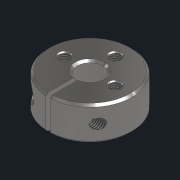
# Autodesk Inventor part: SCSTR6-8b
Saved by Autodesk Inventor 2022 (Build 260153000, 153)
## iProperties
Part Number: SCSTR6-8b
Material: 鋼、炭素鋼
Catalog Web Link: www.cadenas.de
Description: SCST, PSCST, SSCST, SCSTR, PSCSTR, SSCSTR-b-Shaft Collars - 3 Holes/3 Taps
Vendor: MISUMI
Document SubType Name: Modeling
Designer: partserver
Manufacturer: MISUMI
Mass: 15.0833 g
Surface Area: 15.3137 cm^2
Volume: 1.92144 cm^3
Density: 7.85 g/cm^3
Appearance: 半つや出し
Category: PARTsolutions
Company: MISUMI
PSOL_IDENT_0: {$CADENAS_DATA\23d-libs\misumi\metric\03_set_collars\scst\scst_b.prj},209 {VTYP=3D},{NB=SCSTR6-8b},{
PSOL_IDENT_1: LINA=SCSTR6-8},{NN=SCST, PSCST, SSCST, SCSTR, PSCSTR, SSCSTR-b},{DATE=30.06.2021 12:52:04},{GEOMDATE=
PSOL_IDENT_2: 30.10.2015 01:43:51},{VERSION=},{LINEID=220},{WBVAR=TS,MAT,ST,BS},{WBNUMERIC=BS}  {NB=SCSTR6-8b},{LI
PSOL_IDENT_3: NA=SCSTR6-8},{KT=DUMMY},{PN=SCSTR6-8},{TYPE=SCSTR},{TS=3T},{TSALG= '3H' , '3-Hole' , '3T' , '3-Tappe
PSOL_IDENT_4: d' },{TSA= '3H' , '3-Hole', '3T', '3 Tap (Coarse)'},{MAT=S45C},{ST=BO},{STALG= 'BO' , 'Black Oxide'
PSOL_IDENT_5: , 'ENP' , 'Electroless Nickel Plating' },{AC=Hex Socket Head Cap Screw 1 pc.},{ACMAT=4137 Alloy Stee
PSOL_IDENT_6: l},{D=6},{BS=8},{BALG= 8 , 10 },{D1=20},{M=M3},{M3D=3},{DD=3.4},{R=3.00},{W=1.0},{X=6.0},{Y=4},{P=12
PSOL_IDENT_7: },{C=0.5},{S=0.0},{M1=M3},{M13D=3},{L=12}
NB: SCSTR6-8b
NN: SCST, PSCST, SSCST, SCSTR, PSCSTR, SSCSTR-b
NT: Shaft Collars - 3 Holes/3 Taps
NBSYN: $PN.b
LINA: SCSTR6-8
CATALOG: Misumi
PN: SCSTR6-8
TS: 3-Tapped
MAT: 1045 Carbon Steel
ST: Black Oxide
AC: Hex Socket Head Cap Screw 1 pc.
ACMAT: 4137 Alloy Steel
D: 6
BS: 8
D1: 20
M: M3
DD: 3.4
R: 3
W: 1
X: 6
Y: 4
P: 12
C: 0.5
S: 0
M1: M3
SUPPLIER: MISUMI
ARTICLENO: SCSTR6-8b
BOMINFO: SCSTR6-8
CREATOR: CADENAS GmbH
Title: SCSTR6-8
Author: Cadenas PARTsolutions
Comments: Shaft Collars - 3 Holes/3 Taps
Autodesk Inventor part; units mm, degrees
sketch "Sketch_14" plane through (0, 0, 0) normal (1, 0, 0) x (0, 1, 0)
  line L0 (0, -4) -> (0, 4)
  line L1 (0, 4) -> (9.5, 4)
  line L2 (9.5, 4) -> (10, 3.5)
  line L3 (10, 3.5) -> (10, -3.5)
  line L4 (10, -3.5) -> (9.5, -4)
  line L5 (9.5, -4) -> (0, -4)
  line L6 (0, -4) -> (0, 4)
  constraints: 14 end point
revolve "Revolution1" add sketch "Sketch_14" angle 360 about axis through (0, 0, -4) along (0, 0, -1)
sketch "Sketch_15" plane through (0, 0, 0) normal (1, 0, 0) x (0, 1, 0)
  line L0 (0, -4) -> (0, 4)
  line L1 (0, 4) -> (3.5, 4)
  line L2 (3.5, 4) -> (3, 3.5)
  line L3 (3, 3.5) -> (3, -3.5)
  line L4 (3, -3.5) -> (3.5, -4)
  line L5 (3.5, -4) -> (0, -4)
  line L6 (0, -4) -> (0, 4)
  constraints: 14 end point
revolve "Revolution2" cut sketch "Sketch_15" angle 360 about axis through (0, 0, -4) along (0, 0, -1)
sketch "Sketch_16" plane through (0, 0, 0) normal (0, 0, 1) x (1, 0, 0)
  arc A0 (-0.5, -10.9886) -> (0.5, -10.9886) centre (0, 0) ccw
  line L0 (0.5, -10.9886) -> (0.5, 0)
  line L1 (0.5, 0) -> (-0.5, 0)
  line L2 (-0.5, 0) -> (-0.5, -10.9886)
  constraints: 6 end point, 2 point on circle, 1 centre point
extrude "Extrusion1" cut sketch "Sketch_16" along normal mid plane 8
sketch "Sketch_18" plane through (6, 0, 0) normal (1, 0, 0) x (0, 0, -1)
  line L0 (4, 0) -> (-4, 0)
  line L1 (-4, 0) -> (-4, 1.5)
  line L2 (-4, 1.5) -> (-3.7295, 1.2295)
  line L3 (-3.7295, 1.2295) -> (3.7295, 1.2295)
  line L4 (3.7295, 1.2295) -> (4, 1.5)
  line L5 (4, 1.5) -> (4, 0)
  line L6 (4, 0) -> (-4, 0)
  constraints: 14 end point
revolve "Revolution3" cut sketch "Sketch_18" angle 360 about axis through (6, 0, -4) along (0, 0, -1)
thread "Thread1" size "M3x0.5" class "6H" standard "ISO Metric profile" full length
sketch "Sketch_20" plane through (-6, 0, 0) normal (1, 0, 0) x (0, 0, -1)
  line L0 (4, 0) -> (-4, 0)
  line L1 (-4, 0) -> (-4, 1.5)
  line L2 (-4, 1.5) -> (-3.7295, 1.2295)
  line L3 (-3.7295, 1.2295) -> (3.7295, 1.2295)
  line L4 (3.7295, 1.2295) -> (4, 1.5)
  line L5 (4, 1.5) -> (4, 0)
  line L6 (4, 0) -> (-4, 0)
  constraints: 14 end point
revolve "Revolution4" cut sketch "Sketch_20" angle 360 about axis through (-6, 0, -4) along (0, 0, -1)
thread "Thread2" size "M3x0.5" class "6H" standard "ISO Metric profile" full length
sketch "Sketch_22" plane through (0, 6, 0) normal (0, 1, 0) x (1, 0, 0)
  line L0 (0, 4) -> (0, -4)
  line L1 (0, -4) -> (-1.5, -4)
  line L2 (-1.5, -4) -> (-1.2295, -3.7295)
  line L3 (-1.2295, -3.7295) -> (-1.2295, 3.7295)
  line L4 (-1.2295, 3.7295) -> (-1.5, 4)
  line L5 (-1.5, 4) -> (0, 4)
  line L6 (0, 4) -> (0, -4)
  constraints: 14 end point
revolve "Revolution5" cut sketch "Sketch_22" angle 360 about axis through (0, 6, -4) along (0, 0, -1)
thread "Thread3" size "M3x0.5" class "6H" standard "ISO Metric profile" full length
sketch "Sketch_23" plane through (0, -6, 0) normal (0, 1, 0) x (1, 0, 0)
  line L0 (10, 0) -> (0, 0)
  line L1 (0, 0) -> (0, 1.7)
  line L2 (0, 1.7) -> (4, 1.7)
  line L3 (4, 1.7) -> (4, 3)
  line L4 (4, 3) -> (10, 3)
  line L5 (10, 3) -> (10, 0)
  line L6 (10, 0) -> (0, 0)
  constraints: 14 end point
revolve "Revolution6" cut sketch "Sketch_23" angle 360 about axis through (10, -6, 0) along (1, 0, 0)
sketch "Sketch_25" plane through (0, 0, 0) normal (0, 0, 1) x (1, 0, 0)
  line L0 (-0.5, -6) -> (-8.9303, -6)
  line L1 (-8.9303, -6) -> (-8.9303, -4.7705)
  line L2 (-8.9303, -4.7705) -> (-0.7705, -4.7705)
  line L3 (-0.7705, -4.7705) -> (-0.5, -4.5)
  line L4 (-0.5, -4.5) -> (-0.5, -6)
  line L5 (-0.5, -6) -> (-8.9303, -6)
  constraints: 12 end point
revolve "Revolution7" cut sketch "Sketch_25" angle 360 about axis through (-0.5, -6, 0) along (1, 0, 0)
thread "Thread4" size "M3x0.5" class "6H" standard "ISO Metric profile" length 8.1598
ref_plane "to_bolt_XY" through (4, -6, 0) normal (1, 0, 0) x (0, 0, -1)
ref_plane "to_bolt_YZ" through (4, -6, 0) normal (0, 0, -1) x (0, 1, 0)
ref_plane "to_bolt_ZX" through (4, -6, 0) normal (0, 1, 0) x (1, 0, 0)
body "Solid1"
